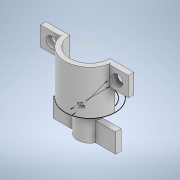
# Autodesk Inventor part: socket
Saved by Autodesk Inventor 2020.2 (Build 242310000, 310)
## iProperties
Created: 2020-02-07
Part Number: socket
Material: Generic
Document SubType Name: Modeling
Designer: ColinP
Density: 1 g/cm^3
Appearance: Default
Author: ColinP
Autodesk Inventor part; units mm, degrees
ref_plane "YZ Plane" through (0, 0, 0) normal (1, 0, 0) x (0, 1, 0)
ref_plane "XZ Plane" through (0, 0, 0) normal (0, 1, 0) x (-1, 0, 0)
ref_plane "XY Plane" through (0, 0, 0) normal (0, 0, 1) x (1, 0, 0)
sketch "Sketch3" plane through (0, 0, 0) normal (0, 1, 0) x (-1, 0, 0)
  circle A0 centre (0, 0) radius 4.5
  circle A1 centre (0, 0) radius 2.6
  dimension "d10" = 9
  dimension "d11" = 5.2
  constraints: 2 centre point, 2 coincident
  measures "d10" diameter of A0
  measures "d11" diameter of A1
extrude "Extrusion2" add sketch "Sketch3" along normal blind 4
sketch "Sketch4" plane through (0, 4, 0) normal (0, 1, 0) x (1, 0, 0)
  circle A0 centre (0, 0) radius 2.6 projected
  line L0 (0, -2.6) -> (0, -1.6)
  line L1 (0, -1.6) -> (0, 2.6)
  line L2 (0, -1.6) -> (-2.0494, -1.6)
  line L3 (0, -1.6) -> (2.0494, -1.6)
  line L4 (0, 2.6) -> (0, 2.6)
  line L5 (0, 2.6) -> (0, 2.6)
  circle A1 centre (0, 0) radius 4.5 projected
  circle A2 centre (0, 0) radius 2.6 projected
  line L6 (0, 2.6) -> (0, 1.6)
  line L7 (0, 1.6) -> (2.0494, 1.6)
  line L8 (0, 1.6) -> (-2.0494, 1.6)
  point P0 (2.0494, 1.6)
  point P1 (-2.0494, 1.6)
  dimension "d14" = 1
  dimension "d20" = 1
  constraints: 18 end point, 7 point on circle, 4 point on line, 1 horizontal, 1 midpoint, 1 parallel, 1 perpendicular, 1 vertical
  measures "d14" distance of L0.start L0.end
  measures "d20" distance of L5.end L6.end
extrude "Extrusion3" add sketch "Sketch4" along normal blind 6 contours L7 L1 A0 | A0 L0 L3 | L1 L8 A0 | A0 L2 L0 | A1
sketch "Sketch5" plane through (0, 10, 0) normal (0, 1, 0) x (1, 0, 0)
  circle A0 centre (0, 0) radius 4.5 projected
extrude "Extrusion4" add sketch "Sketch5" along normal blind 1
sketch "Sketch11" plane through (0, 0, 0) normal (0, -1, 0) x (1, 0, 0)
  point P0 (0, 0)
sketch "Sketch12" plane through (0, 11, 0) normal (0, 1, 0) x (1, 0, 0)
  circle A0 centre (0, 0) radius 7.25
  circle A1 centre (0, 0) radius 9
  dimension "d59" = 14.5
  dimension "d60" = 18
  constraints: 2 centre point, 2 coincident
  measures "d59" diameter of A0
  measures "d60" diameter of A1
extrude "Extrusion11" add sketch "Sketch12" along normal blind 2 contours A0 | A1
extrude "Extrusion12" add sketch "Sketch12" along normal blind 16
sketch "Sketch14" plane through (0, 27, 0) normal (0, 1, 0) x (1, 0, 0)
  point P0 (0, 0)
sketch "Sketch15" plane through (0, 27, 0) normal (0, 1, 0) x (1, 0, 0)
  circle A0 centre (0, 0) radius 9 projected
  line L0 (9, 0) -> (8.9, 0)
  line L1 (8.9, 0) -> (8.9, -1.3379)
  circle A1 centre (0, 0) radius 9 projected
  line L2 (8.9, 0) -> (8.9, 1.3379)
  line L3 (8.9, 1.3379) -> (15.9, 1.3379)
  line L4 (15.9, 1.3379) -> (15.9, -1.3379)
  line L5 (15.9, -1.3379) -> (8.9, -1.3379)
  line L6 (8.9, -1.3379) -> (8.9, 1.3379)
  line L7 (-8.9, 1.3379) -> (-8.9, -1.3379)
  line L8 (-8.9, 1.3379) -> (-15.9, 1.3379)
  line L9 (-15.9, 1.3379) -> (-15.9, -1.3379)
  line L10 (-15.9, -1.3379) -> (-8.9, -1.3379)
  line L11 (-8.9, -1.3379) -> (-8.9, 1.3379)
  dimension "d72" = 0.1
  dimension "d73" = 7
  dimension "d74" = 7
  constraints: 24 end point, 5 point on circle, 4 parallel, 3 horizontal, 3 perpendicular, 2 vertical
  measures "d72" distance of L0.start L0.end
  measures "d73" distance of L4.end L5.end
  measures "d74" distance of L10.end L9.end
extrude "Extrusion14" add sketch "Sketch15" against normal blind 7 contours A0 L3 L4 L5 | A0 L10 L9 L8
sketch "Sketch17" plane through (-8.9, 27, -1.3379) normal (0, 0, -1) x (-1, 0, 0)
  line L0 (7, 0) -> (7, -7) projected
  line L1 (-16.15, 0) -> (7, 0) projected
  line L2 (7, -3.5) -> (3, -3.5)
  line L3 (-24.8, 0) -> (-24.8, -7) projected
  line L4 (-24.8, -3.5) -> (-20.8, -3.5)
  point P0 (-8.9, -27)
  dimension "d81" = 4
  dimension "d82" = 4
  constraints: 4 end point, 2 horizontal, 2 midpoint
  measures "d81" distance of L2.start L2.end
  measures "d82" distance of L4.start L4.end
hole "Hole1" at (-11.9, 23.5, -1.3379) at (11.9, 23.5, -1.3379) direction (0, 0, 1) diameter 3.9 end through all clearance for "Flat Head Machine Screw" size "M3.5" standard "Ansi Metric M Profile"
sketch "Sketch18" plane through (0, 0, 0) normal (0, -1, 0) x (1, 0, 0)
  circle A0 centre (0, 0) radius 4.5 projected
  line L0 (8.9, -1.3379) -> (15.9, -1.3379) projected
  line L1 (4.2982, 1.3326) -> (11.2982, 1.3326)
  line L2 (11.2982, 1.3326) -> (11.2982, -1.3379)
  line L3 (11.2982, -1.3379) -> (4.2982, -1.3379)
  line L4 (4.2982, -1.3379) -> (4.2982, 1.3326)
  circle A1 centre (0, 0) radius 4.5 projected
  line L5 (-4.2982, 1.3326) -> (-11.2982, 1.3326)
  line L6 (-11.2982, 1.3326) -> (-11.2982, -1.3379)
  line L7 (-11.2982, -1.3379) -> (-4.2982, -1.3379)
  line L8 (-4.2982, -1.3379) -> (-4.2982, 1.3326)
  point P0 (4.2982, -1.3326)
  point P1 (-4.2982, -1.3326)
  dimension "d90" = 7
  dimension "d91" = 7
  constraints: 16 end point, 4 parallel, 2 horizontal, 2 perpendicular, 1 point on circle, 1 point on line, 2 other
  measures "d90" distance of L2.end L3.end
  measures "d91" distance of L7.end L6.end
extrude "Extrusion16" add sketch "Sketch18" against normal blind 7 contours A0 L1 L2 L0 L3 | A0 L7 L6 L5
sketch "Sketch19" plane through (4.2982, 0, 1.3326) normal (0, 0, 1) x (1, 0, 0)
  line L0 (7, 0) -> (7, 7) projected
  line L1 (7, 3.5) -> (3.5, 3.5)
  line L2 (-15.5963, 0) -> (-15.5963, 7) projected
  line L3 (-15.5963, 3.5) -> (-12.0963, 3.5)
  point P0 (-4.2982, 0)
  dimension "d94" = 3.5
  dimension "d95" = 3.5
  constraints: 4 end point, 2 horizontal, 2 midpoint
  measures "d94" distance of L1.start L1.end
  measures "d95" distance of L3.start L3.end
hole "Hole2" at (-7.7982, 3.5, 1.3326) at (7.7982, 3.5, 1.3326) direction (0, 0, -1) diameter 3.4 end through all clearance for "Flat Head Machine Screw" size "M3" standard "Ansi Metric M Profile"
sketch "Sketch20" plane through (0, 0, 0) normal (0, -1, 0) x (1, 0, 0)
  line L0 (-15.9, 0) -> (18.3982, 0)
  line L1 (18.3982, 0) -> (18.3982, -9.9107)
  line L2 (18.3982, -9.9107) -> (-15.9, -9.9107)
  line L3 (-15.9, -9.9107) -> (-15.9, 0)
  point P0 (0, 0)
  constraints: 8 end point, 2 parallel, 1 horizontal, 1 perpendicular
extrude "Extrusion17" cut sketch "Sketch20" against normal blind 127
sketch "Sketch21" plane through (11.2982, 0, 0) normal (0, 0, -1) x (-1, 0, 0)
  line L0 (22.5963, 0) -> (22.5963, 7) projected
  line L1 (22.5963, 7) -> (15.7982, 7)
  line L2 (15.7982, 7) -> (15.7982, 0)
  line L3 (15.7982, 0) -> (22.5963, 0)
  line L4 (22.5963, 0) -> (22.5963, 7)
  line L5 (0, 0) -> (7, 0) projected
  line L6 (7, 7) -> (6.7982, 7) projected
  line L7 (0, 0) -> (6.7982, 0)
  line L8 (6.7982, 0) -> (6.7982, 7)
  line L9 (6.7982, 7) -> (0, 7)
  line L10 (0, 7) -> (0, 0)
  line L11 (-4.6018, 20) -> (2.3982, 20) projected
  line L12 (2.3982, 20) -> (2.3982, 27) projected
  line L13 (-4.6018, 20) -> (2.3982, 20)
  line L14 (2.3982, 20) -> (2.3982, 27)
  line L15 (2.3982, 27) -> (-4.6018, 27)
  line L16 (-4.6018, 27) -> (-4.6018, 20)
  line L17 (20.1982, 20) -> (27.1982, 20) projected
  line L18 (20.1982, 27) -> (2.3982, 27) projected
  line L19 (27.1982, 20) -> (20.1982, 20)
  line L20 (20.1982, 20) -> (20.1982, 27)
  line L21 (20.1982, 27) -> (27.1982, 27)
  line L22 (27.1982, 27) -> (27.1982, 20)
  line L23 (18.5482, 27) -> (27.1982, 27) projected
  line L24 (18.5482, 13) -> (18.5482, 27) projected
  line L25 (4.0482, 13) -> (18.5482, 13) projected
  line L26 (4.0482, 27) -> (4.0482, 13) projected
  line L27 (-4.6018, 27) -> (4.0482, 27) projected
  line L28 (-4.6018, 20) -> (-4.6018, 27) projected
  line L29 (2.2982, 20) -> (-4.6018, 20) projected
  line L30 (2.2982, 11) -> (2.2982, 20) projected
  line L31 (6.7982, 11) -> (2.2982, 11) projected
  line L32 (6.7982, 7) -> (6.7982, 11) projected
  line L33 (0, 7) -> (6.7982, 7) projected
  line L34 (0, 0) -> (0, 7) projected
  line L35 (8.6982, 0) -> (0, 0) projected
  line L36 (8.6982, 10) -> (8.6982, 0) projected
  line L37 (13.8982, 10) -> (8.6982, 10) projected
  line L38 (13.8982, 0) -> (13.8982, 10) projected
  line L39 (22.5963, 0) -> (13.8982, 0) projected
  line L40 (22.5963, 7) -> (22.5963, 0) projected
  line L41 (15.7982, 7) -> (22.5963, 7) projected
  line L42 (15.7982, 11) -> (15.7982, 7) projected
  line L43 (20.2982, 11) -> (15.7982, 11) projected
  line L44 (20.2982, 20) -> (20.2982, 11) projected
  line L45 (27.1982, 20) -> (20.2982, 20) projected
  line L46 (27.1982, 27) -> (27.1982, 20) projected
  circle A0 centre (19.0963, 3.5) radius 1.7 projected
  circle A1 centre (3.5, 3.5) radius 1.7 projected
  circle A2 centre (23.1982, 23.5) radius 1.95 projected
  circle A3 centre (-0.6018, 23.5) radius 1.95 projected
  line L47 (15.5963, 0) -> (22.5963, 0) projected
  line L48 (22.5963, 0) -> (15.5963, 0)
  line L49 (15.5963, 0) -> (15.5963, 7)
  line L50 (15.5963, 7) -> (22.5963, 7)
  line L51 (22.5963, 7) -> (22.5963, 0)
  line L52 (7, 0) -> (0, 0)
  line L53 (0, 0) -> (0, 7)
  line L54 (0, 7) -> (7, 7)
  line L55 (7, 7) -> (7, 0)
  line L56 (8.6982, 10) -> (8.6982, 0) projected
  line L57 (0, 0) -> (8.6982, 0)
  line L58 (8.6982, 0) -> (8.6982, 7)
  line L59 (8.6982, 7) -> (0, 7)
  line L60 (0, 7) -> (0, 0)
  line L61 (8.6982, 0) -> (13.8982, 0) projected
  line L62 (13.8982, 0) -> (22.5963, 0)
  line L63 (22.5963, 0) -> (22.5963, 7)
  line L64 (22.5963, 7) -> (13.8982, 7)
  line L65 (13.8982, 7) -> (13.8982, 0)
  point P0 (11.2982, 0)
  constraints: 64 end point, 16 parallel, 8 horizontal, 8 perpendicular, 1 point on line
extrude "Extrusion18" add sketch "Sketch21" against normal blind 2 contours L3 L2 L1 L0 | L39 L49 L50 L2 | L39 L38 L64 L49 | L35 L55 L59 L36 | L17 L20 L21 L22 | L5 L8 L6 L55 | L5 L10 L9 L8 | L12 L11 L16 L15 | A0 | A1
body "Solid2"
